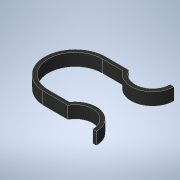
# Autodesk Inventor part: small_belt_loop
Saved by Autodesk Inventor 2021 (Build 250183000, 183)
## iProperties
Created: 2021-02-03
Part Number: small_belt_loop
Material: Generic
Document SubType Name: Modeling
Designer: Jorian Brusind
Density: 1 g/cm^3
Appearance: Rubber - Black
Author: Jorian Brusind
Autodesk Inventor part; units mm, degrees
ref_plane "YZ Plane" through (0, 0, 0) normal (1, 0, 0) x (0, 1, 0)
ref_plane "XZ Plane" through (0, 0, 0) normal (0, 1, 0) x (-1, 0, 0)
ref_plane "XY Plane" through (0, 0, 0) normal (0, 0, 1) x (1, 0, 0)
sketch "Sketch1" plane through (0, 0, 0) normal (0, 1, 0) x (-1, 0, 0)
  arc A0 (-7, 0) -> (7, 0) centre (0, 0) ccw
  line L0 (0, 0) -> (15.4998, -15.4998)
  line L1 (0, 0) -> (21.92, 0) construction
  arc A1 (14.3592, -26.1891) -> (7.8984, -7.8984) centre (15.4998, -15.4998) ccw
  line L2 (0, 0) -> (-7, 0)
  line L3 (15.4998, -15.4998) -> (15.4998, -4.7498)
  line L4 (15.4998, -15.4998) -> (26.2498, -15.4998) construction
  line L5 (15.4998, -4.7498) -> (5.1419, -4.7498)
  line L6 (15.4998, -15.4998) -> (15.4998, -26.2498)
  line L7 (15.4998, -15.4998) -> (37.4198, -15.4998) construction
  line L8 (15.4998, -26.2498) -> (26.0213, -26.2498) construction
  arc A2 (14.7522, -27.727) -> (16.2473, -3.2726) centre (15.4998, -15.4998) ccw
  line L9 (15.4998, -15.4998) -> (14.7522, -27.727) construction
  line L10 (15.4998, -15.4998) -> (16.2473, -3.2726) construction
  line L11 (-8.5, 0) -> (-7, 0)
  arc A3 (-8.5, 0) -> (7.0336, -4.7726) centre (0, 0) ccw
  line L12 (0, 0) -> (-8.5, 0) construction
  line L13 (0, 0) -> (8.5, 0) construction
  line L14 (7.0336, -4.7726) -> (7.0336, -3.2726)
  line L15 (7.0336, -3.2726) -> (6.1879, -3.2726)
  line L16 (7.0336, -3.2726) -> (16.2473, -3.2726)
  line L17 (14.7522, -27.727) -> (22.4821, -27.727) construction
  line L18 (15.4998, -15.4998) -> (0, -15.4998)
  line L19 (15.4998, -15.4998) -> (0, -30.9996)
  line L20 (15.4998, -15.4998) -> (37.4198, -15.4998) construction
  line L21 (14.3592, -26.1891) -> (22.4791, -26.1891) construction
  arc A4 (7, -30.9996) -> (-7, -30.9996) centre (0, -30.9996) ccw
  arc A5 (8.6, -30.9996) -> (-8.6, -30.9996) centre (0, -30.9996) ccw
  line L22 (15.4998, -26.2498) -> (7.1694, -26.2498)
  line L23 (14.7522, -27.727) -> (7.953, -27.727)
  line L24 (-8.6, -30.9996) -> (-7, -30.9996)
  line L25 (7.953, -27.727) -> (6.1879, -27.727)
  dimension "d0" = 14
  dimension "d1" = 21.92
  dimension "d2" = 45
  dimension "d3" = 21.5
  dimension "d4" = 10.75
  dimension "d5" = 90
  dimension "d6" = 90
  dimension "d13" = 12.25
  dimension "d14" = 180
  dimension "d21" = 8.5
  dimension "d22" = 180
  dimension "d23" = 1.5
  dimension "d24" = 90
  dimension "d25" = 7.0336
  dimension "d31" = 21.92
  dimension "d32" = 135
  dimension "d44" = 7
  dimension "d45" = 8.6
  constraints: 52 end point, 18 point on circle, 14 horizontal, 6 centre point, 6 coincident, 4 equal length, 3 point on line, 3 vertical, 2 parallel, 1 tangent
  measures "d0" diameter of A0
  measures "d1" distance of L0.start L0.end
  measures "d2" angle of L0 L1
  measures "d3" diameter of A1
  measures "d4" distance of L3.start L3.end
  measures "d5" angle of L4 L3
  measures "d6" angle of L5 L3
  measures "d13" radius of A2
  measures "d14" angle of L9 L10
  measures "d21" radius of A3
  measures "d22" angle of L12 L13
  measures "d23" distance of L14.start L14.end
  measures "d24" angle of L15 L14
  measures "d25" distance from line of L0.start L14
  measures "d31" distance of L9.start L19.end
  measures "d32" angle of L19 L20
  measures "d44" radius of A4
  measures "d45" radius of A5
extrude "Extrusion3" add sketch "Sketch1" along normal blind 5 contours L5 L14 A3 L0 A0 | A0 L15 L14 L5 | L0 A3 L11 A0 | L14 L16 A2 L23 A5 L22 A1 L5 | A1 L6 L3 | A5 L25 A4 L19 | L19 A4 L24 A5
sketch "Sketch3" plane through (0, 5, 0) normal (0, 1, 0) x (1, 0, 0)
  line L0 (-15.4998, 26.2498) -> (-15.4998, 4.7498) projected
  arc A0 (-15.4998, 26.2498) -> (-15.4998, 4.7498) centre (-15.4998, 15.4998) ccw
  line L1 (-15.4998, 4.7498) -> (-15.4998, 15.4998)
  line L2 (-15.4998, 15.4998) -> (-15.4998, 26.2498)
  point P0 (0, 0)
  constraints: 4 end point, 2 collinear, 2 point on circle, 1 centre point, 1 midpoint
extrude "Extrusion4" cut sketch "Sketch3" against normal blind 5
body "Solid2"
